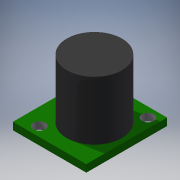
# Autodesk Inventor part: SONIC
Saved by Autodesk Inventor 2019 (Build 230136000, 136)
## iProperties
Created: 2020-03-15
Part Number: SONIC
Material: Generic
Document SubType Name: Modeling
Designer: Pulag
Density: 1 g/cm^3
Appearance: Default
Author: Pulag
Autodesk Inventor part; units mm, degrees
ref_plane "YZ Plane" through (0, 0, 0) normal (1, 0, 0) x (0, 1, 0)
ref_plane "XZ Plane" through (0, 0, 0) normal (0, 1, 0) x (-1, 0, 0)
ref_plane "XY Plane" through (0, 0, 0) normal (0, 0, 1) x (1, 0, 0)
sketch "Sketch1" plane through (0, 0, 0) normal (0, 1, 0) x (-1, 0, 0)
  line L0 (-10, 11) -> (10, 11)
  line L1 (10, 11) -> (10, -11)
  line L2 (10, -11) -> (-10, -11)
  line L3 (-10, -11) -> (-10, 11)
  line L4 (-10, 11) -> (10, -11) construction
  line L5 (10, 11) -> (-10, -11) construction
  point P0 (0, 0)
  dimension "d0" = 20
  dimension "d1" = 22
  constraints: 12 end point, 2 midpoint, 2 parallel, 1 horizontal, 1 perpendicular
  measures "d0" distance of L1.end L2.end
  measures "d1" distance of L0.end L1.end
extrude "Extrusion1" add sketch "Sketch1" against normal blind 2
sketch "Sketch2" plane through (0, 0, 0) normal (0, 1, 0) x (1, 0, 0)
  circle A0 centre (1.2, 0) radius 7.5
  line L0 (-10, 11) -> (10, 11) projected
  line L1 (10, -11) -> (10, 11)
  dimension "d4" = 15
  dimension "d10" = 8.8
  constraints: 2 end point, 1 centre point, 1 vertical
  measures "d4" diameter of A0
  measures "d10" distance from line of A0.centre L1
extrude "Extrusion2" add sketch "Sketch2" along normal blind 16
sketch "Sketch3" plane through (0, 0, 0) normal (0, 1, 0) x (1, 0, 0)
  line L0 (-10, -8.4) -> (-10, -11)
  circle A0 centre (-5.4, -8.4) radius 1.6
  circle A1 centre (7.4, 8.4) radius 1.6
  point P0 (0, 0)
  point P1 (10, 11)
  dimension "d9" = 3.2
  dimension "d13" = 3.2
  constraints: 2 centre point, 2 end point
  measures "d9" diameter of A0
  measures "d13" diameter of A1
extrude "Extrusion3" cut sketch "Sketch3" against normal up to surface (2 mm away)
body "Solid1"
